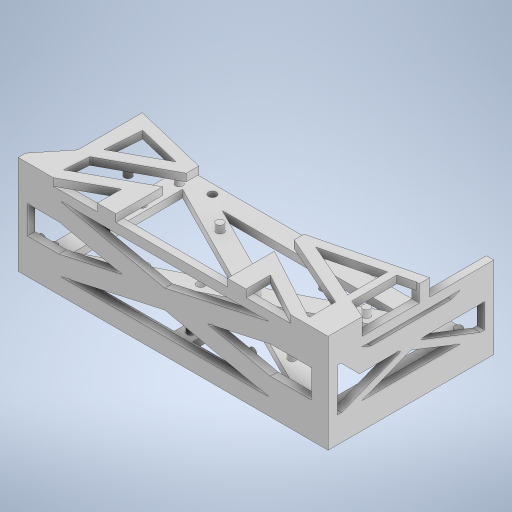
# Autodesk Inventor part: Power_Supply
Saved by Autodesk Inventor 2024 (Build 280153000, 153)
## iProperties
Created: 2024-11-22
Part Number: Power_Supply
Material: Generic
Document SubType Name: Modeling
Designer: Owner
Density: 1 g/cm^3
Appearance: Default
Author: Owner
Autodesk Inventor part; units mm, degrees
ref_plane "YZ Plane" through (0, 0, 0) normal (1, 0, 0) x (0, 1, 0)
ref_plane "XZ Plane" through (0, 0, 0) normal (0, 1, 0) x (-1, 0, 0)
ref_plane "XY Plane" through (0, 0, 0) normal (0, 0, 1) x (1, 0, 0)
sketch "Sketch1" plane through (0, 0, 0) normal (0, 1, 0) x (-1, 0, 0)
  line L0 (88.9, 50.8) -> (-88.9, 50.8)
  line L1 (-88.9, 50.8) -> (-88.9, -50.8)
  line L2 (-88.9, -50.8) -> (88.9, -50.8)
  line L3 (88.9, -50.8) -> (88.9, 50.8)
  line L4 (88.9, 50.8) -> (-88.9, -50.8) construction
  line L5 (-88.9, 50.8) -> (88.9, -50.8) construction
  point P0 (0, 0)
  dimension "d0" = 177.8
  dimension "d1" = 101.6
  constraints: 12 end point, 2 midpoint, 2 parallel, 1 horizontal, 1 perpendicular
  measures "d0" distance of L2.end L1.end
  measures "d1" distance of L1.end L0.end
extrude "Extrusion1" add sketch "Sketch1" along normal blind 44.45
sketch "Sketch2" plane through (-88.9, 0, 50.8) normal (0, 0, 1) x (1, 0, 0)
  line L0 (177.8, 0) -> (177.8, 44.45) projected
  line L1 (177.8, 44.45) -> (184.15, 44.45)
  line L2 (184.15, 44.45) -> (184.15, 0)
  line L3 (184.15, 0) -> (177.8, 0)
  line L4 (177.8, 0) -> (177.8, 44.45)
  line L5 (177.8, 44.45) -> (0, 44.45) projected
  line L6 (0, 44.45) -> (-15.875, 44.45)
  line L7 (-15.875, 44.45) -> (-15.875, 0)
  line L8 (-15.875, 0) -> (0, 0)
  line L9 (0, 0) -> (0, 44.45)
  point P0 (88.9, 0)
  dimension "d4" = 6.35
  dimension "d5" = 15.875
  constraints: 16 end point, 4 parallel, 2 horizontal, 2 perpendicular, 1 point on line
  measures "d4" distance of L2.end L3.end
  measures "d5" distance of L8.end L7.end
extrude "Extrusion2" add sketch "Sketch2" against normal blind 1.5875
sketch "Sketch3" plane through (0, 0, 0) normal (0, -1, 0) x (1, 0, 0)
  line L0 (-104.775, 49.2125) -> (-88.9, 49.2125) projected
  line L1 (-88.9, -50.8) -> (-88.9, 49.2125) projected
  line L2 (-104.775, 49.2125) -> (-88.9, 49.2125)
  line L3 (-88.9, 49.2125) -> (-88.9, -50.8)
  line L4 (-88.9, -50.8) -> (-104.775, -50.8)
  line L5 (-104.775, -50.8) -> (-104.775, 49.2125)
  line L6 (88.9, 49.2125) -> (95.25, 49.2125) projected
  line L7 (95.25, 49.2125) -> (88.9, 49.2125)
  line L8 (88.9, 49.2125) -> (88.9, -50.8)
  line L9 (88.9, -50.8) -> (95.25, -50.8)
  line L10 (95.25, -50.8) -> (95.25, 49.2125)
  point P0 (0, 0)
  constraints: 16 end point, 4 parallel, 2 horizontal, 2 perpendicular, 1 point on line
extrude "Extrusion3" add sketch "Sketch3" against normal blind 1.5875
sketch "Sketch4" plane through (0, 1.5875, 0) normal (0, 1, 0) x (1, 0, 0)
  line L0 (88.9, -49.2125) -> (95.25, -49.2125) projected
  line L1 (95.25, -50.8) -> (95.25, 50.8) projected
  line L2 (88.9, -49.2125) -> (95.25, -49.2125)
  line L3 (95.25, -49.2125) -> (95.25, 36.5125)
  line L4 (95.25, 36.5125) -> (88.9, 36.5125)
  line L5 (88.9, 36.5125) -> (88.9, -49.2125)
  point P0 (0, 0)
  dimension "d10" = 85.725
  constraints: 8 end point, 2 parallel, 1 horizontal, 1 perpendicular, 1 point on line
  measures "d10" distance of L3.end L2.end
extrude "Extrusion4" add sketch "Sketch4" along normal blind 12.7
sketch "Sketch5" plane through (-104.775, 0, 50.8) normal (0, 0, 1) x (1, 0, 0)
  line L0 (200.025, 44.45) -> (0, 44.45) projected
  line L1 (200.025, 0) -> (200.025, 44.45) projected
  line L2 (0, 44.45) -> (200.025, 0)
  line L3 (200.025, 0) -> (200.025, 44.45)
  line L4 (0, 0) -> (200.025, 0) projected
  line L5 (200.025, 44.45) -> (0, 0)
  line L6 (100.0125, 44.45) -> (100.0125, 0)
  line L7 (0, 44.45) -> (0, 0) projected
  line L8 (0, 22.225) -> (200.025, 22.225)
  line L9 (100.0125, 22.225) -> (0, 22.225)
  line L10 (100.0125, 22.225) -> (200.025, 22.225)
  line L11 (6.35, 6.35) -> (193.675, 6.35)
  line L12 (193.675, 6.35) -> (193.675, 38.1)
  line L13 (193.675, 38.1) -> (6.35, 38.1)
  line L14 (6.35, 38.1) -> (6.35, 6.35)
  line L15 (6.35, 6.35) -> (193.675, 38.1) construction
  line L16 (193.675, 6.35) -> (6.35, 38.1) construction
  circle A0 centre (6.35, 38.1) radius 2.54
  circle A1 centre (6.35, 6.35) radius 2.54
  circle A2 centre (100.0125, 22.225) radius 2.54
  circle A3 centre (193.675, 6.35) radius 2.54
  circle A4 centre (193.675, 38.1) radius 2.54
  line L17 (100.0125, 22.225) -> (0, 22.225)
  line L18 (50.0063, 22.225) -> (50.0063, 44.45)
  line L19 (50.0063, 22.225) -> (50.0063, 0)
  line L20 (100.0125, 22.225) -> (200.025, 22.225)
  line L21 (150.0188, 22.225) -> (150.0188, 44.45)
  line L22 (150.0188, 22.225) -> (150.0188, 0)
  circle A5 centre (50.0063, 33.3375) radius 2.54
  circle A6 centre (50.0063, 11.1125) radius 2.54
  circle A7 centre (150.0188, 11.1125) radius 2.54
  circle A8 centre (150.0188, 33.3375) radius 2.54
  point P0 (104.775, 0)
  dimension "d13" = 187.325
  dimension "d14" = 31.75
  dimension "d15" = 5.08
  dimension "d16" = 5.08
  dimension "d17" = 5.08
  dimension "d18" = 5.08
  dimension "d19" = 5.08
  dimension "d20" = 5.08
  dimension "d21" = 5.08
  dimension "d22" = 5.08
  dimension "d23" = 5.08
  constraints: 38 end point, 13 midpoint, 9 centre point, 6 point on line, 5 coincident, 4 collinear, 4 perpendicular, 2 parallel, 1 horizontal
  measures "d13" distance of L13.end L12.end
  measures "d14" distance of L12.end L11.end
  measures "d15" diameter of A0
  measures "d16" diameter of A1
  measures "d17" diameter of A2
  measures "d18" diameter of A3
  measures "d19" diameter of A4
  measures "d20" diameter of A5
  measures "d21" diameter of A6
  measures "d22" diameter of A7
  measures "d23" diameter of A8
extrude "Extrusion5" add sketch "Sketch5" along normal blind 6.35 contours A8 L21 L5 | L5 L21 A8 | A4 L12 L13 | L13 L12 A4 | L21 L5 A8 | A3 L11 L12 | L12 L11 A3 | L21 A8 L5 | A2 L5 L6 | L6 L2 A2 | A7 L22 L2 | L2 L22 A7 | A2 L2 L8 | L8 L5 A2 | L22 L2 A7 | A5 L2 L18 | L18 L2 A5 | L8 A2 L2 | L6 A2 L5 | L2 A2 L6 | L5 A2 L8 | L22 A7 L2 | L2 L18 A5 | A0 L14 L13 | L13 L14 A0 | L2 A5 L18 | A1 L11 L14 | L14 L11 A1 | A6 L19 L5 | L5 L19 A6 | A6 L5 L19 | A6 L19 L5
sketch "Sketch6" plane through (0, 44.45, 0) normal (0, 1, 0) x (1, 0, 0)
  line L0 (88.9, -49.2125) -> (88.9, 50.8) projected
  line L1 (88.9, 50.8) -> (-88.9, 50.8)
  line L2 (-88.9, 50.8) -> (-88.9, -50.8)
  line L3 (-88.9, -50.8) -> (88.9, -50.8)
  line L4 (88.9, -50.8) -> (88.9, 50.8)
  line L5 (-88.9, 0) -> (-88.9, -50.8)
  line L6 (-88.9, 0) -> (88.9, 0)
  line L7 (88.9, -50.8) -> (88.9, 0)
  line L8 (-88.9, 50.8) -> (-88.9, -49.2125) projected
  line L9 (-88.9, -25.4) -> (88.9, -25.4)
  line L10 (0, 0) -> (0, -50.8)
  line L11 (0, 0) -> (-88.9, 0)
  line L12 (0, 0) -> (88.9, 0)
  line L13 (-44.45, 0) -> (-44.45, -50.8)
  line L14 (44.45, 0) -> (44.45, -50.8)
  line L15 (-104.775, -50.8) -> (95.25, -50.8) projected
  line L16 (-88.9, 0) -> (88.9, -50.8)
  line L17 (-88.9, -50.8) -> (88.9, 0)
  circle A0 centre (-44.45, -12.7) radius 2.54
  circle A1 centre (44.45, -12.7) radius 2.54
  circle A2 centre (44.45, -38.1) radius 2.54
  circle A3 centre (-44.45, -38.1) radius 2.54
  line L18 (-88.9, -25.4) -> (-44.45, -25.4)
  circle A4 centre (-66.675, -25.4) radius 2.54
  line L19 (44.45, -25.4) -> (88.9, -25.4)
  circle A5 centre (66.675, -25.4) radius 2.54
  dimension "d26" = 5.08
  dimension "d27" = 5.08
  dimension "d28" = 5.08
  dimension "d29" = 5.08
  dimension "d30" = 5.08
  dimension "d31" = 5.08
  constraints: 34 end point, 11 point on line, 10 midpoint, 6 centre point, 3 collinear, 3 parallel, 3 perpendicular, 1 horizontal
  measures "d26" diameter of A0
  measures "d27" diameter of A1
  measures "d28" diameter of A2
  measures "d29" diameter of A3
  measures "d30" diameter of A4
  measures "d31" diameter of A5
extrude "Extrusion6" add sketch "Sketch6" along normal blind 6.35 contours A5 L9 | L9 A5 | A2 L14 L16 | L16 L14 A2 | A1 L14 L17 | L17 L14 A1 | A2 L16 L14 | L16 A2 L14 | L14 L17 A1 | L14 A1 L17 | A3 L17 L13 | L13 L17 A3 | A0 L13 L16 | L16 L13 A0 | L17 L13 A3 | A0 L13 L16 | L16 L13 A0 | A3 L13 L17 | A4 L9 | L9 A4
sketch "Sketch7" plane through (88.9, 44.45, 49.2125) normal (1, 0, 0) x (0, 0, -1)
  line L0 (0, -30.1625) -> (85.725, -30.1625) projected
  line L1 (85.725, -30.1625) -> (100.0125, -30.1625)
  line L2 (100.0125, -42.8625) -> (100.0125, 0) projected
  line L3 (0, 0) -> (100.0125, 0)
  line L4 (100.0125, 0) -> (100.0125, -30.1625)
  line L5 (100.0125, -30.1625) -> (0, -30.1625)
  line L6 (0, -30.1625) -> (0, 0)
  line L7 (0, -15.0813) -> (100.0125, -15.0813)
  line L8 (50.0062, 0) -> (50.0062, -30.1625)
  line L9 (50.0062, -15.0813) -> (0, -15.0813)
  line L10 (-1.5875, 0) -> (-1.5875, -44.45) projected
  line L11 (25.0031, -15.0813) -> (0, -15.0813)
  line L12 (12.5016, -15.0813) -> (12.5016, 0)
  line L13 (8.5725, 0) -> (13.6525, 0) projected
  line L14 (12.5016, -15.0813) -> (12.5016, -30.1625)
  line L15 (50.0062, -15.0813) -> (100.0125, -15.0813)
  line L16 (75.0094, -15.0813) -> (100.0125, -15.0813)
  line L17 (87.5109, -15.0813) -> (100.0125, -15.0813)
  line L18 (87.5109, -15.0813) -> (87.5109, 0)
  line L19 (87.5109, -15.0813) -> (87.5109, -30.1625)
  circle A0 centre (12.5016, -15.0813) radius 2.54
  circle A1 centre (50.0062, -15.0813) radius 2.54
  circle A2 centre (87.5109, -15.0813) radius 2.54
  point P0 (49.2125, -44.45)
  dimension "d34" = 5.08
  dimension "d35" = 5.08
  dimension "d36" = 5.08
  constraints: 32 end point, 9 midpoint, 7 point on line, 5 perpendicular, 3 centre point, 3 coincident, 3 collinear, 2 horizontal, 2 parallel
  measures "d34" diameter of A0
  measures "d35" diameter of A1
  measures "d36" diameter of A2
extrude "Extrusion7" add sketch "Sketch7" along normal blind 12.7 contours A0 L7 L14 | L14 L7 A0 | A0 L12 L7 | A1 L7 L8 | L8 L7 A1 | L12 A0 L7 | L8 A1 L7 | L7 A1 L8 | A2 L7 L19 | L19 L7 A2 | L18 A2 L7 | L7 A2 L18
sketch "Sketch8" plane through (-98.425, 6.35, 57.15) normal (0, 0, 1) x (1, 0, 0)
  line L0 (-6.35, 38.1) -> (9.525, 38.1) projected
  line L1 (-6.35, -6.35) -> (193.675, -6.35) projected
  line L2 (-6.35, 38.1) -> (193.675, 38.1)
  line L3 (193.675, 38.1) -> (193.675, -6.35)
  line L4 (193.675, -6.35) -> (-6.35, -6.35)
  line L5 (-6.35, -6.35) -> (-6.35, 38.1)
  line L6 (193.675, -6.35) -> (-6.35, 38.1)
  line L7 (193.675, 38.1) -> (-6.35, -6.35)
  line L8 (195.0525, 31.9012) -> (-4.9725, -12.5488)
  line L9 (192.2975, 44.2988) -> (-7.7275, -0.1512)
  line L10 (195.0525, -0.1512) -> (-4.9725, 44.2988)
  line L11 (192.2975, -12.5488) -> (-7.7275, 31.9012)
  point P0 (98.425, -6.35)
  point P1 (122.9346, 15.875)
  point P2 (193.675, 31.5951)
  point P3 (164.4029, 38.1)
  point P4 (93.6625, 22.3799)
  point P5 (22.9221, 38.1)
  point P6 (-6.35, 31.5951)
  point P7 (64.3904, 15.875)
  point P8 (-6.35, 0.1549)
  point P9 (22.9221, -6.35)
  point P10 (93.6625, 9.3701)
  point P11 (164.4029, -6.35)
  point P12 (193.675, 0.1549)
  dimension "d95" = 6.35
  dimension "d96" = 6.35
  dimension "d97" = 6.35
  dimension "d98" = 6.35
  constraints: 20 end point, 6 parallel, 1 horizontal, 1 perpendicular
  measures "d95" distance between parallel lines of L7 L8
  measures "d96" distance between parallel lines of L7 L9
  measures "d97" distance between parallel lines of L6 L10
  measures "d98" distance between parallel lines of L6 L11
extrude "Extrusion8" add sketch "Sketch8" along normal blind 5.08 contours L6 L9 L11 L5 | L0 L2 L10 L9 L6 | L9 L10 L7 L6 | L6 L7 L11 L9 | L9 L11 L7 L5 | L7 L10 L8 L6 | L6 L8 L11 L7 | L9 L2 L7 L10 | L7 L11 L8 L1 | L8 L10 L3 L6 | L6 L1 L11 L8 | L7 L3 L8 L10
sketch "Sketch9" plane through (101.6, 29.3688, -0.7937) normal (1, 0, 0) x (0, 0, -1)
  line L0 (-63.0237, 15.0813) -> (-63.0237, -29.3688) projected
  line L1 (-63.0237, 15.0813) -> (50.0063, 15.0813)
  line L2 (50.0063, 15.0813) -> (50.0063, -29.3688)
  line L3 (50.0063, -29.3688) -> (-63.0237, -29.3688)
  line L4 (-63.0237, -29.3688) -> (-63.0237, 15.0813)
  line L5 (50.0063, -29.3688) -> (-63.0237, 15.0813)
  line L6 (-63.0237, -29.3688) -> (-63.0237, 15.0813) projected
  line L7 (-63.0237, -29.3688) -> (50.0063, 15.0813)
  line L8 (-63.9533, -27.005) -> (49.0767, 17.445)
  line L9 (-62.0942, -31.7325) -> (50.9358, 12.7175)
  line L10 (49.0767, -31.7325) -> (-63.9533, 12.7175)
  line L11 (50.9358, -27.005) -> (-62.0942, 17.445)
  circle A0 centre (0, 0) radius 2.54 projected
  line L12 (0, 0) -> (50.0063, 0)
  line L13 (0, 0) -> (-63.0237, 0)
  line L14 (-63.0237, 6.35) -> (0, 6.35)
  line L15 (0, 6.35) -> (50.0063, 6.35)
  line L16 (-63.0237, -6.35) -> (0, -6.35)
  line L17 (0, -6.35) -> (50.0063, -6.35)
  line L18 (43.6563, 8.7312) -> (-56.6737, 8.7312)
  line L19 (-56.6737, 8.7312) -> (-56.6737, -23.0187)
  line L20 (-56.6737, -23.0187) -> (43.6563, -23.0187)
  line L21 (43.6563, -23.0187) -> (43.6563, 8.7312)
  line L22 (43.6563, 8.7312) -> (-56.6737, -23.0187) construction
  line L23 (-56.6737, 8.7312) -> (43.6563, -23.0187) construction
  line L24 (-56.6737, 8.7312) -> (-41.5925, -6.35)
  line L25 (-56.6737, 8.7312) -> (-35.3456, 8.7312) construction
  point P0 (-0.7937, -29.3688)
  point P1 (-6.5087, -7.1437)
  point P2 (-39.9363, -23.0187)
  point P3 (-6.5087, -9.8731)
  point P4 (26.9188, -23.0187)
  point P5 (-15.4675, -6.35)
  point P6 (-13.4491, -7.1437)
  point P7 (-53.817, -23.0187)
  point P8 (-56.6737, 6.35)
  point P9 (-54.2925, 6.35)
  point P10 (0.4316, -7.1437)
  point P11 (2.45, -6.35)
  point P12 (43.6563, -6.35)
  point P13 (40.7995, -23.0187)
  point P14 (-33.8811, 6.35)
  point P15 (-39.9363, 8.7312)
  point P16 (26.9188, 8.7312)
  point P17 (20.8636, 6.35)
  dimension "d86" = 2.54
  dimension "d87" = 2.54
  dimension "d88" = 2.54
  dimension "d89" = 2.54
  dimension "d90" = 6.35
  dimension "d91" = 6.35
  dimension "d92" = 100.33
  dimension "d93" = 31.75
  dimension "d94" = 45
  constraints: 48 end point, 8 parallel, 4 point on line, 3 horizontal, 3 midpoint, 3 perpendicular, 1 equal length, 2 other
  measures "d86" distance between parallel lines of L7 L8
  measures "d87" distance between parallel lines of L7 L9
  measures "d88" distance between parallel lines of L5 L10
  measures "d89" distance between parallel lines of L5 L11
  measures "d90" distance between parallel lines of L13 L14
  measures "d91" distance between parallel lines of L13 L16
  measures "d92" distance of L20.end L19.end
  measures "d93" distance of L19.end L18.end
  measures "d94" angle of L24 L25
extrude "Extrusion9" add sketch "Sketch9" along normal blind 5.08 contours L14 L19 L13 L0 | L0 L10 L18 L19 L14 | L13 L19 L16 L0 | L0 L5 L18 L10 | L19 L24 L14 | L16 L19 L20 L8 L0 | L1 L11 L18 L5 | L18 L5 L14 L10 | L10 L14 L24 L18 | L14 L10 L13 L24 | L8 L20 L7 L0 | L13 L10 L16 L24 | L1 L8 L18 L11 | L18 L11 L14 L5 | L14 L5 L13 L10 | L7 L20 L9 L3 | L8 L10 L7 L20 | L13 L5 L8 L16 L10 | L1 L7 L18 L8 | L14 L11 L13 L5 | L9 L20 L10 L3 | L7 L10 L9 L20 | L10 L16 L8 | L8 L16 L5 L7 L10 | L13 L11 L8 L5 | L2 L9 L18 L7 | L18 L7 L15 L8 | L14 L15 L8 L12 A0 L13 L11 | L10 L20 L5 L3 | L7 L5 L9 L10 | L8 L5 L16 | L8 L11 L7 L16 L5 | L13 A0 L8 L11 | L2 L15 L21 L18 L9 | L18 L9 L15 L7 | L15 L7 L12 L8 | L5 L20 L11 L2 | L10 L9 L5 L20 | L7 L16 L11 L9 L5 | L5 L16 L7 | L8 A0 L12 L7 L11 | L13 L12 A0 L8 | A0 L12 L13 | L2 L12 L21 L15 | L18 L21 L15 L9 | L15 L9 L12 L7 | L8 A0 L12 | L11 L20 L21 L17 L2 | L5 L9 L11 L20 | L7 L11 L16 | L8 A0 | L7 L12 L9 L17 L16 L11 | L2 L17 L21 L12 | L21 L12 L9 L15 | L11 L16 L17 L9 | L21 L17 L9 L12
sketch "Sketch10" plane through (-44.45, 50.8, 12.7) normal (0, 1, 0) x (1, 0, 0)
  line L0 (151.13, 63.5) -> (151.13, -49.53) projected
  line L1 (-60.325, -44.45) -> (-60.325, -49.53) projected
  line L2 (151.13, 63.5) -> (-60.325, 63.5)
  line L3 (-60.325, 63.5) -> (-60.325, -49.53)
  line L4 (-60.325, -49.53) -> (151.13, -49.53)
  line L5 (151.13, -49.53) -> (151.13, 63.5)
  line L6 (-60.325, -38.1) -> (-60.325, 63.5) projected
  line L7 (-60.325, 12.7) -> (151.13, 12.7)
  line L8 (151.13, 12.7) -> (151.13, -49.53)
  line L9 (151.13, -49.53) -> (-60.325, -49.53)
  line L10 (-60.325, -49.53) -> (-60.325, 12.7)
  line L11 (-44.45, 63.5) -> (-44.45, -36.5125) projected
  circle A0 centre (0, 0) radius 2.54 projected
  line L12 (0, 0) -> (6.333, 0.4643)
  line L13 (6.333, 0.4643) -> (6.333, 12.7)
  line L14 (6.333, 0.4643) -> (6.333, -49.53)
  line L15 (-44.45, 12.7) -> (6.333, 0.4643)
  line L16 (133.35, -36.5125) -> (133.35, 49.2125) projected
  circle A1 centre (88.9, 0) radius 2.54 projected
  line L17 (88.9, 0) -> (82.55, 0)
  line L18 (82.55, 0) -> (82.55, 12.7)
  line L19 (82.55, 0) -> (82.55, -38.1)
  line L20 (82.55, -38.1) -> (133.35, -38.1)
  line L21 (82.55, -38.1) -> (133.35, -38.1)
  line L22 (151.13, 17.145) -> (82.55, 0)
  line L23 (-44.224, 15.2582) -> (6.6826, 2.9927)
  line L24 (151.13, 19.7632) -> (81.934, 2.4642)
  line L25 (-44.45, 12.7) -> (-44.45, -49.53)
  line L26 (-44.45, -49.53) -> (6.333, -49.53)
  line L27 (82.55, -38.1) -> (82.55, -49.53)
  line L28 (82.55, -49.53) -> (151.13, -49.53)
  line L29 (6.6826, 2.9927) -> (-44.45, -24.765)
  circle A2 centre (0, -25.4) radius 2.54 projected
  line L30 (-44.45, -49.53) -> (0, -25.4)
  line L31 (0, -25.4) -> (6.333, -21.9621)
  line L32 (-46.2677, -21.4166) -> (-3.8484, 1.6111)
  line L33 (-3.8484, 1.6111) -> (-45.1165, 11.5542)
  line L34 (-44.45, -29.1002) -> (17.2137, 4.3744)
  line L35 (17.2137, 4.3744) -> (-44.45, 19.2317)
  line L36 (-46.2677, -46.1816) -> (6.333, -17.6269)
  line L37 (-1.8177, -22.0516) -> (4.5153, -18.6137)
  line L38 (-42.6323, -52.8784) -> (1.8177, -28.7484)
  line L39 (1.8177, -28.7484) -> (8.1507, -25.3105)
  line L40 (0, -25.4) -> (-6.35, -25.4)
  line L41 (-6.35, -25.4) -> (-6.35, -49.53)
  circle A3 centre (111.125, -12.7) radius 2.54 projected
  line L42 (82.55, 0) -> (111.125, -12.7)
  line L43 (111.125, -12.7) -> (151.13, -30.48)
  line L44 (84.0974, 3.4816) -> (112.6724, -9.2184)
  line L45 (112.6724, -9.2184) -> (152.6774, -26.9984)
  line L46 (151.13, -34.6493) -> (109.5776, -16.1816)
  line L47 (109.5776, -16.1816) -> (81.0026, -3.4816)
  line L48 (-60.325, -49.53) -> (-44.45, -24.765)
  line L49 (-44.45, -49.53) -> (-38.1, -49.53)
  line L50 (-38.1, -49.53) -> (-33.6063, 12.7)
  circle A4 centre (88.9, -25.4) radius 2.54 projected
  line L51 (82.55, -21.9621) -> (88.9, -25.4)
  line L52 (88.9, -25.4) -> (133.4693, -49.53)
  line L53 (141.4717, -49.53) -> (90.714, -22.0495)
  line L54 (90.714, -22.0495) -> (82.55, -17.6295)
  line L55 (131.6553, -52.8805) -> (87.086, -28.7505)
  line L56 (87.086, -28.7505) -> (80.736, -25.3126)
  line L57 (152.0541, 13.4488) -> (83.4741, -3.6962)
  line L58 (146.05, -49.53) -> (151.13, -49.53) projected
  line L59 (151.13, -49.53) -> (138.43, -49.53)
  line L60 (138.43, -49.53) -> (138.43, 12.7)
  line L61 (133.4693, -49.53) -> (133.35, 12.7)
  line L62 (88.9, -25.4) -> (95.25, -25.4)
  line L63 (68.9596, -44.45) -> (131.7015, -44.45) projected
  line L64 (95.25, -25.4) -> (95.25, -49.53)
  line L65 (-44.45, 19.2317) -> (-44.45, 12.7)
  point P0 (44.45, 12.7)
  point P1 (6.333, 2.8029)
  point P2 (6.333, 3.077)
  point P3 (6.333, 6.996)
  point P4 (-17.3409, 12.7)
  point P5 (-36.4641, -49.53)
  point P6 (-6.35, -33.1823)
  point P7 (-6.35, -49.53)
  point P8 (-44.45, -45.1948)
  point P9 (-44.45, -36.5125)
  point P10 (6.333, -1.5323)
  point P11 (-44.45, -20.4298)
  point P12 (-44.45, 11.3937)
  point P13 (133.35, -18.4084)
  point P14 (94.2091, -1.0125)
  point P15 (133.35, 8.7727)
  point P16 (82.55, -4.1693)
  point P17 (138.43, -29.0049)
  point P18 (138.43, -47.8832)
  point P19 (82.55, -49.53)
  point P20 (82.55, 2.6182)
  point P21 (133.4257, -26.7808)
  point P22 (133.461, -45.1929)
  point P23 (95.25, -49.53)
  point P24 (95.25, -33.1705)
  point P25 (125.4668, -49.53)
  point P26 (151.13, -26.3107)
  point P27 (138.43, -20.6662)
  point P28 (138.43, 10.0427)
  point P29 (149.059, 12.7)
  point P30 (-37.5151, -41.4301)
  point P31 (-36.3055, -24.6789)
  point P32 (-35.6539, -15.6548)
  point P33 (-33.8845, 8.848)
  dimension "d106" = 6.35
  dimension "d107" = 6.35
  dimension "d108" = 2.54
  dimension "d109" = 2.54
  dimension "d110" = 3.81
  dimension "d111" = 3.81
  dimension "d112" = 3.81
  dimension "d113" = 3.81
  dimension "d114" = 6.35
  dimension "d115" = 3.81
  dimension "d116" = 3.81
  dimension "d117" = 6.35
  dimension "d118" = 3.81
  dimension "d119" = 3.81
  dimension "d120" = 3.81
  dimension "d121" = 12.7
  dimension "d122" = 6.35
  constraints: 118 end point, 33 point on line, 10 perpendicular, 9 parallel, 4 collinear, 4 horizontal, 1 midpoint, 4 other
  measures "d106" distance of L12.start L12.end
  measures "d107" distance of L17.start L17.end
  measures "d108" distance between parallel lines of L15 L23
  measures "d109" distance between parallel lines of L22 L24
  measures "d110" distance between parallel lines of L29 L32
  measures "d111" distance between parallel lines of L29 L34
  measures "d112" distance between parallel lines of L30 L36
  measures "d113" distance between parallel lines of L30 L38
  measures "d114" distance of L30.end L40.end
  measures "d115" distance between parallel lines of L42 L44
  measures "d116" distance between parallel lines of L43 L46
  measures "d117" distance of L25.end L49.end
  measures "d118" distance between parallel lines of L52 L53
  measures "d119" distance between parallel lines of L52 L55
  measures "d120" distance between parallel lines of L22 L57
  measures "d121" distance of L0.end L59.end
  measures "d122" distance of L51.end L62.end
extrude "Extrusion10" add sketch "Sketch10" along normal blind 5.08 contours L0 L22 L16 L24 | L0 L57 L7 L22 | L16 L7 L24 | L35 L7 L11 | L0 L7 L57 | L22 A1 L44 L24 L7 | L61 L57 L16 | L16 L57 L44 A1 L22 | L7 L60 L57 L61 | L15 L50 L33 L11 | L7 L50 L15 | L35 L13 L23 L7 | L57 L60 L7 | L57 L61 L45 L16 | L22 L44 A1 | A1 L44 L22 | L57 L60 L45 L61 | L44 A1 L22 L18 L24 | L23 L13 L29 L15 A0 L50 | L33 L50 L32 L11 | L15 A0 L29 L50 L32 L33 | L0 L43 L60 L45 | L45 L61 L43 L16 | L16 L43 A3 L42 L57 A1 L44 L45 | L57 A1 L44 | A1 L57 L22 L44 | L44 L22 A1 | L45 L60 L43 L61 | L32 L50 L29 L11 | L15 A0 L29 | A0 L15 | L0 L46 L60 L43 | L43 L61 L46 L16 | L16 L46 L47 L19 L42 A3 L43 | A1 L57 | A1 L17 L22 | L43 L60 L46 L61 | L17 A1 L57 L42 | L48 L11 L25 L4 | L13 L15 L29 | L29 L50 L34 L11 | L15 L29 A0 | L29 L12 A0 | A0 L12 L14 L34 L50 L29 | L0 L4 L53 L60 L46 | L43 L42 A3 | A3 L42 L43 | L46 L60 L53 L61 | L30 L50 L4 | L25 L36 L50 L30 | L12 A0 L29 L15 | L34 L50 L36 L25 L11 | A0 L12 L29 | L14 L31 A2 L40 L41 L30 L50 L36 | L61 L52 L20 L53 | L53 L60 L4 L61 | L54 L53 L20 L52 L64 L62 A4 L51 L19 | L50 L30 L41 L38 L4 | L14 L39 L38 L41 L30 A2 L31 | L53 L4 L60 | L4 L55 L63 L52 | L51 A4 L52 L64 L55 L56 L19 | L41 L40 A2 L30 | L14 L4 L41 L38 L39 | L31 L40 A2 | A2 L30 L31 | L52 L63 L55 L20 | L20 L55 L64 L52 | L56 L55 L64 L20 L19 | L51 L52 A4 | A4 L62 L51 | A2 L40 L30 | L52 A4 L62 L64 | L4 L27 L63 L64 | L20 L64 L63 L27 | A4 L52 L62
sketch "Sketch11" plane through (-104.775, 0, 57.15) normal (-1, 0, 0) x (0, 0, 1)
  line L0 (0, 0) -> (0, 44.45) projected
  line L1 (0, 44.45) -> (0, 50.8)
  line L2 (5.08, 50.8) -> (-64.2132, 50.8) projected
  line L3 (-107.95, 44.45) -> (5.08, 44.45) projected
  line L4 (0, 50.8) -> (5.08, 50.8)
  line L5 (5.08, 50.8) -> (5.08, 44.45)
  line L6 (5.08, 44.45) -> (0, 44.45)
  line L7 (0, 44.45) -> (0, 50.8)
  point P0 (-57.15, 0)
  point P1 (-57.15, 50.8)
  constraints: 10 end point, 2 parallel, 1 horizontal, 1 perpendicular, 1 point on line, 1 vertical
extrude "Extrusion11" add sketch "Sketch11" against normal up to surface (211.455 mm away)
sketch "Sketch12" plane through (101.6, 44.45, 57.15) normal (0, -1, 0) x (1, 0, 0)
  line L0 (-6.35, 0) -> (-6.35, 5.08) projected
  line L1 (-6.35, 5.08) -> (0, 5.08) projected
  line L2 (-6.35, 0) -> (0, 0)
  line L3 (0, 0) -> (0, 5.08)
  line L4 (0, 5.08) -> (-6.35, 5.08)
  line L5 (-6.35, 5.08) -> (-6.35, 0)
  point P0 (-101.6, -57.15)
  constraints: 8 end point, 2 parallel, 1 horizontal, 1 perpendicular
extrude "Extrusion12" add sketch "Sketch12" along normal up to surface (44.45 mm away)
sketch "Sketch13" plane through (-98.425, 6.35, 57.15) normal (0, 0, -1) x (-1, 0, 0)
  line L0 (-200.025, 38.1) -> (-205.105, 38.1) projected
  line L1 (-200.025, 38.1) -> (-200.025, 44.45)
  line L2 (-205.105, 44.45) -> (3.0936, 44.45) projected
  line L3 (-205.105, 44.45) -> (-205.105, 38.1) projected
  line L4 (-200.025, 44.45) -> (-205.105, 44.45)
  line L5 (-205.105, 44.45) -> (-205.105, 38.1)
  line L6 (-205.105, 38.1) -> (-200.025, 38.1)
  line L7 (-200.025, 38.1) -> (-200.025, 44.45)
  point P0 (-98.425, -6.35)
  point P1 (6.35, 44.45)
  constraints: 10 end point, 2 parallel, 1 horizontal, 1 perpendicular, 1 point on line, 1 vertical
extrude "Extrusion13" add sketch "Sketch13" along normal up to surface (57.15 mm away)
sketch "Sketch14" plane through (0, 0, 0) normal (0, -1, 0) x (1, 0, 0)
  line L0 (95.25, 50.8) -> (95.25, -50.8) projected
  line L1 (95.25, 50.8) -> (-104.775, 50.8) projected
  line L2 (95.25, -50.8) -> (-104.775, -50.8)
  line L3 (-104.775, -50.8) -> (-104.775, 50.8)
  line L4 (-104.775, 50.8) -> (95.25, 50.8)
  line L5 (95.25, 50.8) -> (95.25, -50.8)
  line L6 (-104.775, -50.8) -> (95.25, -50.8) projected
  line L7 (-4.7625, -50.8) -> (-4.7625, 50.8)
  line L8 (104.609, 0) -> (106.68, 0) projected
  line L9 (95.25, 0) -> (-104.775, 0)
  line L10 (88.9, 44.45) -> (-98.425, 44.45)
  line L11 (-98.425, 44.45) -> (-98.425, -44.45)
  line L12 (-98.425, -44.45) -> (88.9, -44.45)
  line L13 (88.9, -44.45) -> (88.9, 44.45)
  line L14 (88.9, 44.45) -> (-98.425, -44.45) construction
  line L15 (-98.425, 44.45) -> (88.9, -44.45) construction
  line L16 (95.25, -50.8) -> (-104.775, 50.8)
  line L17 (95.25, 50.8) -> (-104.775, -50.8)
  line L18 (95.25, 0) -> (-4.7625, 0)
  line L19 (45.2438, 0) -> (45.2438, -50.8)
  line L20 (45.2438, 0) -> (45.2438, 44.45)
  line L21 (-4.7625, 0) -> (-104.775, 0)
  line L22 (-54.7688, 0) -> (-54.7688, -44.45)
  line L23 (-54.7688, 0) -> (-54.7688, 50.8)
  circle A0 centre (-4.7625, 0) radius 2.54
  circle A1 centre (-54.7688, -25.4) radius 2.54
  circle A2 centre (-54.7688, 25.4) radius 2.54
  circle A3 centre (45.2438, 25.4) radius 2.54
  circle A4 centre (45.2438, -25.4) radius 2.54
  circle A5 centre (88.9, -44.45) radius 2.54
  circle A6 centre (88.9, 44.45) radius 2.54
  circle A7 centre (-98.425, 44.45) radius 2.54
  circle A8 centre (-98.425, -44.45) radius 2.54
  circle A9 centre (-4.7625, 44.45) radius 2.54
  circle A10 centre (-4.7625, -44.45) radius 2.54
  point P0 (0, 0)
  point P1 (101.6, 0)
  point P2 (-4.7625, 46.99)
  point P3 (-4.7625, 44.45)
  point P4 (-7.3025, 44.45)
  point P5 (-61.7909, 0)
  dimension "d51" = 187.325
  dimension "d52" = 88.9
  dimension "d53" = 5.08
  dimension "d54" = 5.08
  dimension "d55" = 5.08
  dimension "d56" = 5.08
  dimension "d57" = 5.08
  dimension "d58" = 5.08
  dimension "d59" = 5.08
  dimension "d60" = 5.08
  dimension "d61" = 5.08
  dimension "d62" = 5.08
  dimension "d63" = 5.08
  constraints: 40 end point, 12 midpoint, 11 centre point, 10 point on line, 5 coincident, 4 parallel, 4 perpendicular, 3 collinear, 2 horizontal
  measures "d51" distance of L12.end L11.end
  measures "d52" distance of L11.end L10.end
  measures "d53" diameter of A0
  measures "d54" diameter of A1
  measures "d55" diameter of A2
  measures "d56" diameter of A3
  measures "d57" diameter of A4
  measures "d58" diameter of A5
  measures "d59" diameter of A6
  measures "d60" diameter of A7
  measures "d61" diameter of A8
  measures "d62" diameter of A9
  measures "d63" diameter of A10
extrude "Extrusion14" add sketch "Sketch14" along normal blind 6.35 contours A9 L10 L7 | L7 L10 A9 | A6 L13 L10 | L10 L13 A6 | A3 L20 L17 | L17 L20 A3 | A5 L12 L13 | L13 L12 A5 | L10 A9 L7 | L7 A9 L10 | L20 L17 A3 | L20 A3 L17 | A4 L19 L16 | L16 L19 A4 | A0 L16 L9 | L9 L17 A0 | L19 L16 A4 | A2 L16 L23 | L23 L16 A2 | A10 L12 L7 | L7 L12 A10 | L12 L7 A10 | A4 L16 L19 | L16 A0 L7 | L16 A0 L7 | L17 A0 L9 | L9 A0 L16 | L7 A0 L17 | L7 A0 L17 | A7 L11 L10 | L10 L11 A7 | L16 L23 A2 | L16 A2 L23 | L12 A10 L7 | A8 L12 L11 | L11 L12 A8 | A1 L22 L17 | L17 L22 A1 | A1 L22 L17 | L17 L22 A1
sketch "Sketch15" plane through (88.9, -6.35, -44.45) normal (0, -1, 0) x (1, 0, 0)
  line L0 (-193.675, 106.68) -> (17.78, 106.68) projected
  line L1 (-193.675, 106.68) -> (17.78, 106.68)
  line L2 (17.78, 106.68) -> (17.78, -6.35)
  line L3 (17.78, -6.35) -> (-193.675, -6.35)
  line L4 (-193.675, -6.35) -> (-193.675, 106.68)
  line L5 (0, -6.35) -> (-6.35, -6.35)
  line L6 (0, -6.35) -> (-177.8, -6.35) projected
  line L7 (-6.35, -6.35) -> (17.78, -6.35)
  line L8 (17.78, -6.35) -> (17.78, 106.68)
  line L9 (17.78, 106.68) -> (-6.35, 106.68)
  line L10 (-6.35, 106.68) -> (-6.35, -6.35)
  line L11 (-193.675, -6.35) -> (6.35, -6.35) projected
  line L12 (-193.675, -6.35) -> (-180.975, -6.35)
  line L13 (-180.975, -6.35) -> (-180.975, 106.68)
  line L14 (-180.975, 106.68) -> (-193.675, 106.68)
  line L15 (-193.675, 106.68) -> (-193.675, -6.35)
  line L16 (6.35, -6.35) -> (-193.675, 95.25)
  line L17 (6.35, 95.25) -> (-193.675, -6.35)
  line L18 (3.4743, -12.0115) -> (-196.5507, 89.5885)
  line L19 (9.2257, -0.6885) -> (-190.7993, 100.9115)
  line L20 (9.2257, 89.5885) -> (-190.7993, -12.0115)
  line L21 (3.4743, 100.9115) -> (-196.5507, -0.6885)
  line L22 (17.78, 106.68) -> (-193.675, 106.68)
  line L23 (-193.675, 106.68) -> (-193.675, 93.98)
  line L24 (-193.675, 93.98) -> (17.78, 93.98)
  line L25 (17.78, 93.98) -> (17.78, 106.68)
  line L26 (17.78, -6.35) -> (-193.675, -6.35)
  line L27 (-193.675, -6.35) -> (-193.675, 6.35)
  line L28 (-193.675, 6.35) -> (17.78, 6.35)
  line L29 (17.78, 6.35) -> (17.78, -6.35)
  point P0 (-88.9, 44.45)
  point P1 (-79.6407, 44.45)
  point P2 (-6.35, 81.677)
  point P3 (-6.35, 7.223)
  point P4 (-93.6625, 37.3278)
  point P5 (-32.6749, 6.35)
  point P6 (-154.6501, 6.35)
  point P7 (-107.6843, 44.45)
  point P8 (-180.975, 7.223)
  point P9 (-180.975, 81.677)
  point P10 (-10.1721, 93.98)
  point P11 (-93.6625, 51.5722)
  point P12 (-177.1529, 93.98)
  dimension "d72" = 6.35
  dimension "d73" = 12.7
  dimension "d74" = 6.35
  dimension "d75" = 6.35
  dimension "d76" = 6.35
  dimension "d77" = 6.35
  dimension "d78" = 12.7
  dimension "d79" = 12.7
  constraints: 54 end point, 14 parallel, 5 horizontal, 5 perpendicular, 5 point on line
  measures "d72" distance of L5.start L5.end
  measures "d73" distance of L14.end L13.end
  measures "d74" distance between parallel lines of L16 L18
  measures "d75" distance between parallel lines of L16 L19
  measures "d76" distance between parallel lines of L17 L20
  measures "d77" distance between parallel lines of L17 L21
  measures "d78" distance of L23.end L22.end
  measures "d79" distance of L26.end L27.end
extrude "Extrusion15" add sketch "Sketch15" along normal blind 5.08 contours L0 L13 L24 L16 L4 | L0 L10 L21 L24 L19 L13 | L16 L24 L4 | L0 L2 L24 L10 | L19 L24 L13 | L24 L16 L13 L18 L4 | L24 L13 L16 | L10 L24 L21 | L24 L19 L21 L16 L13 | L18 L13 L21 L28 L4 | L16 L21 L18 L13 | L2 L28 L19 L10 L17 L24 | L24 L17 L10 | L10 L17 L19 L21 L24 | L19 L17 L16 L21 | L28 L21 L4 | L16 L17 L18 L21 | L2 L3 L16 L10 L28 | L10 L20 L19 L17 | L19 L20 L16 L17 | L21 L28 L13 L17 L4 | L21 L13 L28 | L21 L18 L17 L28 L13 | L16 L20 L18 L17 | L28 L10 L19 | L19 L10 L28 L16 L20 | L17 L13 L3 | L28 L17 L13 | L18 L20 L28 L17 | L16 L28 L18 L20 | L3 L10 L16 | L10 L16 L28 | L13 L17 L28 L20 L3 | L16 L10 L3 L18 L28 | L20 L28 L18 L3
sketch "Sketch16" plane through (106.68, -6.35, 62.23) normal (1, 0, 0) x (0, 0, -1)
  line L0 (0, 6.35) -> (0, 62.23) projected
  line L1 (113.03, 0) -> (0, 0) projected
  line L2 (0, 6.35) -> (113.03, 6.35)
  line L3 (113.03, 6.35) -> (113.03, 0)
  line L4 (113.03, 0) -> (0, 0)
  line L5 (0, 0) -> (0, 6.35)
  point P0 (62.23, 6.35)
  constraints: 8 end point, 2 parallel, 1 horizontal, 1 perpendicular
extrude "Extrusion16" add sketch "Sketch16" against normal up to surface (5.08 mm away)
sketch "Sketch17" plane through (101.6, 29.3688, -0.7937) normal (-1, 0, 0) x (0, 0, 1)
  line L0 (57.9437, -29.3688) -> (63.0237, -29.3688) projected
  line L1 (57.9437, -29.3688) -> (57.9437, -35.7188)
  line L2 (63.0238, -35.7188) -> (-50.0063, -35.7188) projected
  line L3 (63.0238, -35.7188) -> (63.0237, -29.3688) projected
  line L4 (57.9437, -29.3688) -> (63.0238, -29.3688)
  line L5 (63.0238, -29.3688) -> (63.0238, -35.7188)
  line L6 (63.0238, -35.7188) -> (57.9437, -35.7188)
  line L7 (57.9437, -35.7188) -> (57.9437, -29.3688)
  point P0 (0.7937, -29.3688)
  constraints: 10 end point, 2 parallel, 1 horizontal, 1 perpendicular, 1 point on line, 1 vertical
extrude "Extrusion17" add sketch "Sketch17" along normal up to surface (206.375 mm away)
sketch "Sketch18" plane through (88.9, -11.43, -44.45) normal (0, -1, 0) x (1, 0, 0)
  circle A0 centre (-93.6625, 88.9) radius 2.54 projected
  line L0 (-93.6625, 88.9) -> (-93.6625, 93.98)
  line L1 (-177.1529, 93.98) -> (-10.1721, 93.98) projected
  line L2 (-93.6625, 93.98) -> (-87.3125, 93.98)
  line L3 (-93.6625, 88.9) -> (-93.6625, 82.55)
  line L4 (-93.6625, 82.55) -> (-100.0125, 82.55)
  line L5 (-87.3125, 93.98) -> (-100.0125, 93.98)
  line L6 (-100.0125, 93.98) -> (-100.0125, 82.55)
  line L7 (-100.0125, 82.55) -> (-87.3125, 82.55)
  line L8 (-87.3125, 82.55) -> (-87.3125, 93.98)
  point P0 (-88.9, 44.45)
  dimension "d80" = 6.35
  dimension "d81" = 6.35
  dimension "d82" = 6.35
  constraints: 16 end point, 2 parallel, 2 perpendicular, 1 horizontal, 1 midpoint, 1 point on line, 1 vertical
  measures "d80" distance of L0.end L2.end
  measures "d81" distance of L0.start L3.end
  measures "d82" distance of L3.end L4.end
extrude "Extrusion18" add sketch "Sketch18" against normal up to surface (5.08 mm away)
fillet "Fillet1" radius 3.175 2 edges at (-11.1125, -8.89, 38.1) (1.5875, -8.89, 38.1)
sketch "Sketch19" plane through (-104.775, 0, 57.15) normal (0, 0, 1) x (1, 0, 0)
  circle A0 centre (193.675, 38.1) radius 2.54 projected
  line L0 (193.675, 38.1) -> (193.675, 31.75)
  line L1 (193.675, 44.45) -> (193.675, 14.2875) projected
  circle A1 centre (193.675, 6.35) radius 2.54 projected
  line L2 (193.675, 6.35) -> (193.675, 12.7)
  line L3 (193.675, 1.5875) -> (193.675, 44.45) projected
  line L4 (193.675, 12.7) -> (200.025, 12.7)
  line L5 (200.025, 1.5875) -> (200.025, 14.2875) projected
  line L6 (193.675, 12.7) -> (172.1471, 12.7)
  line L7 (192.0265, 8.2824) -> (129.2846, 22.225) projected
  line L8 (193.675, 31.75) -> (200.025, 31.75)
  line L9 (200.025, 31.75) -> (172.1471, 31.75)
  line L10 (129.2846, 22.225) -> (200.025, 37.9451) projected
  line L11 (172.1471, 31.75) -> (200.025, 37.9451)
  line L12 (200.025, 37.9451) -> (200.025, 31.75)
  line L13 (200.025, 6.5049) -> (129.2846, 22.225) projected
  line L14 (172.1471, 12.7) -> (200.025, 6.5049)
  line L15 (200.025, 6.5049) -> (200.025, 12.7)
  circle A2 centre (6.35, 38.1) radius 2.54 projected
  line L16 (6.35, 38.1) -> (6.35, 31.75)
  line L17 (6.35, 31.75) -> (0, 31.75)
  line L18 (0, 44.45) -> (0, 0) projected
  line L19 (0, 38.1) -> (0, 31.75)
  line L20 (6.35, 31.75) -> (27.8779, 31.75)
  line L21 (7.9985, 36.1676) -> (70.7404, 22.225) projected
  line L22 (0, 37.9451) -> (4.0382, 37.0477) projected
  line L23 (0, 37.9451) -> (27.8779, 31.75)
  circle A3 centre (6.35, 6.35) radius 2.54 projected
  line L24 (6.35, 6.35) -> (6.35, 12.7)
  line L25 (6.35, 12.7) -> (0, 12.7)
  line L26 (0, 12.7) -> (27.8779, 12.7)
  line L27 (27.8779, 12.7) -> (0, 6.5049)
  line L28 (0, 6.5049) -> (0, 12.7)
  point P0 (104.775, 0)
  dimension "d99" = 6.35
  dimension "d100" = 6.35
  dimension "d101" = 6.35
  dimension "d102" = 6.35
  constraints: 40 end point, 17 point on line, 4 collinear, 3 perpendicular, 1 horizontal, 1 parallel, 1 other
  measures "d99" distance of L0.start L0.end
  measures "d100" distance of L2.start L2.end
  measures "d101" distance of L16.start L16.end
  measures "d102" distance of L24.start L24.end
extrude "Extrusion19" add sketch "Sketch19" along normal blind 5.08 contours L10 L12 L8 L0 A0 | A0 L0 L10 | L10 L0 A0 | A0 L0 L9 L10 | L6 L2 A1 L7 | L4 L5 L13 A1 L2 | A1 L2 L13 | A1 L13 L2 | L23 L16 A2 | A2 L16 L17 L18 L22 | L21 L20 L16 A2 | A2 L16 L23 | L25 L24 A3 L27 L18 | L26 L27 A3 L24 | A3 L24 L27 | A3 L27 L24
sketch "Sketch20" plane through (106.68, 50.8, -7.0632) normal (1, 0, 0) x (0, 0, -1)
  line L0 (0, 0) -> (-17.145, 0) projected
  line L1 (43.7368, -6.35) -> (-56.2757, -6.35) projected
  line L2 (0, 0) -> (-7.0632, 0)
  line L3 (-7.0632, 0) -> (-7.0632, -6.35)
  line L4 (-7.0632, -6.35) -> (0, -6.35)
  line L5 (0, -6.35) -> (0, 0)
  point P0 (-7.0632, -50.8)
  point P1 (0, -6.35)
  constraints: 8 end point, 2 parallel, 1 horizontal, 1 perpendicular, 1 point on line
extrude "Extrusion20" add sketch "Sketch20" against normal up to surface (5.08 mm away)
sketch "Sketch21" plane through (101.6, 50.8, -7.0632) normal (0, 1, 0) x (1, 0, 0)
  line L0 (5.08, 0) -> (-63.5, -17.145) projected
  line L1 (0, -1.27) -> (0, 0) projected
  line L2 (5.08, 0) -> (0, -1.27)
  line L3 (0, -1.27) -> (0, 0)
  line L4 (0, -1.27) -> (0, 0)
  line L5 (0, 0) -> (5.08, 0) projected
  line L6 (5.08, 0) -> (0, 0)
  point P0 (-101.6, -7.0632)
  constraints: 8 end point, 2 collinear, 1 vertical
extrude "Extrusion21" cut sketch "Sketch21" against normal up to surface (6.35 mm away)
sketch "Sketch22" plane through (-104.775, -6.35, -50.8) normal (-1, 0, 0) x (0, 0, 1)
  line L0 (101.6, 50.8) -> (100.0125, 50.8) projected
  line L1 (0, 6.35) -> (101.6, 6.35)
  line L2 (101.6, 6.35) -> (101.6, 50.8)
  line L3 (101.6, 50.8) -> (0, 50.8)
  line L4 (0, 50.8) -> (0, 6.35)
  line L5 (0, 28.575) -> (101.6, 28.575)
  line L6 (50.8, 6.35) -> (50.8, 50.8)
  line L7 (102.87, 5.08) -> (-1.27, 5.08)
  line L8 (-1.27, 5.08) -> (-1.27, 52.07)
  line L9 (-1.27, 52.07) -> (102.87, 52.07)
  line L10 (102.87, 52.07) -> (102.87, 5.08)
  line L11 (102.87, 5.08) -> (-1.27, 52.07) construction
  line L12 (-1.27, 5.08) -> (102.87, 52.07) construction
  point P0 (50.8, 28.575)
  dimension "d127" = 104.14
  dimension "d128" = 46.99
  constraints: 24 end point, 6 midpoint, 4 parallel, 2 horizontal, 2 perpendicular
  measures "d127" distance of L8.end L9.end
  measures "d128" distance of L7.end L8.end
extrude "Extrusion22" cut sketch "Sketch22" against normal blind 194.945 contours L2 L5 L6 L3 L0 | L2 L1 L6 L5 | L6 L5 L4 L3 | L6 L1 L4 L5 | L7 L8 L9 L10
sketch "Sketch23" plane through (90.17, -6.35, -50.8) normal (-1, 0, 0) x (0, 0, 1)
  line L0 (0, -5.08) -> (0, 50.8) projected
  line L1 (0, 6.35) -> (101.4986, 6.35)
  line L2 (101.4986, 6.35) -> (101.4986, 50.8)
  line L3 (101.4986, 50.8) -> (0, 50.8)
  line L4 (0, 50.8) -> (0, 6.35)
  line L5 (102.7686, 5.08) -> (-1.27, 5.08)
  line L6 (-1.27, 5.08) -> (-1.27, 52.07)
  line L7 (-1.27, 52.07) -> (102.7686, 52.07)
  line L8 (102.7686, 52.07) -> (102.7686, 5.08)
  line L9 (-1.27, 28.575) -> (102.7686, 28.575)
  line L10 (94.0747, 52.07) -> (89.9498, 5.08)
  line L11 (89.9498, 5.08) -> (102.7686, 5.08)
  line L12 (102.7686, 52.07) -> (102.7686, 5.08)
  line L13 (102.7686, 52.07) -> (94.0747, 52.07)
  point P0 (50.8, 6.35)
  point P1 (92.0122, 28.575)
  dimension "d131" = 1.27
  constraints: 26 end point, 4 parallel, 3 perpendicular, 3 point on line, 2 collinear, 2 midpoint, 1 horizontal, 3 other
  measures "d131" distance between parallel lines of L1 L5
extrude "Extrusion23" cut sketch "Sketch23" against normal up to surface (11.43 mm away) contours L5 L6 L9 L0 | L0 L1 L10 L5 | L0 L9 L10 L1 | L10 L1 L2 L9 L8 L5 | L10 L9 L2 L1 | L10 L3 L2 L9 | L9 L2 L3 L10 L7 L8
sketch "Sketch24" plane through (-98.425, 6.35, 62.23) normal (0, 0, 1) x (1, 0, 0)
  line L0 (-6.35, 6.35) -> (-6.35, -12.7) projected
  line L1 (-6.35, 25.4) -> (21.5279, 25.4) projected
  line L2 (-6.35, 6.35) -> (0, 6.35)
  line L3 (0, 6.35) -> (0, 25.4)
  line L4 (0, 25.4) -> (-6.35, 25.4)
  line L5 (-6.35, 25.4) -> (-6.35, 6.35)
  point P0 (98.425, -6.35)
  dimension "d134" = 6.35
  constraints: 8 end point, 2 parallel, 1 horizontal, 1 perpendicular, 1 point on line
  measures "d134" distance of L4.end L3.end
extrude "Extrusion24" add sketch "Sketch24" against normal up to surface (5.08 mm away)
sketch "Sketch25" plane through (88.9, -6.35, -44.45) normal (0, 1, 0) x (1, 0, 0)
  line L0 (-32.6749, -6.35) -> (-154.6501, -6.35) projected
  line L1 (-154.6501, -6.35) -> (-193.675, -6.35)
  line L2 (-193.675, -101.6) -> (-193.675, 6.35) projected
  line L3 (-93.6625, -37.3278) -> (-32.6749, -6.35) projected
  line L4 (-32.6749, -6.35) -> (12.7, -6.35)
  line L5 (12.7, -101.6) -> (12.7, 6.35) projected
  line L6 (-193.675, 6.35) -> (12.7, 6.35) projected
  line L7 (-193.675, -6.35) -> (12.7, -6.35)
  line L8 (12.7, -6.35) -> (12.7, 6.35)
  line L9 (12.7, 6.35) -> (-193.675, 6.35)
  line L10 (-193.675, 6.35) -> (-193.675, -6.35)
  line L11 (-193.675, 0) -> (12.7, 0)
  line L12 (-6.35, -81.677) -> (-6.35, -7.223) projected
  line L13 (-6.35, -7.223) -> (-6.35, -6.35)
  line L14 (-32.6749, -6.35) -> (-6.35, -6.35)
  line L15 (-19.5125, -6.35) -> (-19.5125, 6.35)
  line L16 (-180.975, -7.223) -> (-180.975, -81.677) projected
  line L17 (-180.975, -7.223) -> (-180.975, -6.35)
  line L18 (-180.975, -6.35) -> (-154.6501, -6.35)
  line L19 (-167.8125, -6.35) -> (-167.8125, 6.35)
  circle A0 centre (-167.8125, 0) radius 2.667
  circle A1 centre (-19.5125, 0) radius 2.667
  circle A2 centre (-93.6625, -44.45) radius 2.54 projected
  circle A3 centre (-143.6687, -69.85) radius 2.54 projected
  line L20 (-93.6625, -44.45) -> (-143.6687, -69.85)
  circle A4 centre (-43.6562, -69.85) radius 2.54 projected
  line L21 (-93.6625, -44.45) -> (-43.6562, -69.85)
  circle A5 centre (-118.6656, -57.15) radius 2.667
  circle A6 centre (-68.6594, -57.15) radius 2.667
  point P0 (-88.9, -44.45)
  dimension "d137" = 5.334
  dimension "d138" = 5.334
  dimension "d139" = 5.334
  dimension "d140" = 5.334
  constraints: 30 end point, 8 midpoint, 7 point on line, 4 centre point, 4 perpendicular, 2 collinear, 2 horizontal, 2 parallel, 1 vertical
  measures "d137" diameter of A0
  measures "d138" diameter of A1
  measures "d139" diameter of A5
  measures "d140" diameter of A6
extrude "Extrusion25" cut sketch "Sketch25" against normal blind 25.4 contours A1 L11 L15 | L15 L11 A1 | A0 L11 L19 | L19 L11 A0 | L15 A1 L11 | L11 A1 L15 | L19 A0 L11 | L11 A0 L19 | A5 L20 | L20 A5 | A6 L21 | L21 A6
sketch "Sketch26" plane through (-44.45, 55.88, 12.7) normal (0, 1, 0) x (1, 0, 0)
  line L0 (-60.325, -44.45) -> (146.05, -44.45) projected
  line L1 (-44.45, -24.765) -> (-57.0686, -44.45) projected
  line L2 (-60.325, -44.45) -> (-44.45, -24.765)
  line L3 (-60.325, -49.53) -> (-36.4641, -49.53) projected
  line L4 (-44.45, -24.765) -> (-60.325, -49.53)
  line L5 (-60.325, -49.53) -> (-60.325, -44.45)
  point P0 (44.45, 12.7)
  constraints: 6 end point, 1 point on line, 1 vertical
extrude "Extrusion26" add sketch "Sketch26" against normal up to surface (5.08 mm away)
sketch "Sketch27" plane through (87.6387, 50.8, 57.15) normal (0, 1, 0) x (1, 0, 0)
  line L0 (0, 0) -> (1.3708, 0) projected
  line L1 (0, 0) -> (1.3708, 0)
  line L2 (1.3723, -0.7429) -> (-49.5387, 26.8205) projected
  line L3 (1.3708, 0) -> (1.3723, -0.7429)
  line L4 (1.3723, -0.7429) -> (0, 0)
  point P0 (-87.6387, 57.15)
  constraints: 6 end point, 1 collinear, 1 horizontal
extrude "Extrusion27" add sketch "Sketch27" along normal up to surface (5.08 mm away)
sketch "Sketch28" plane through (106.68, 29.3688, -0.7937) normal (1, 0, 0) x (0, 0, -1)
  line L0 (6.2694, 15.0813) -> (6.2694, 26.5113) projected
  line L1 (6.2694, 15.0813) -> (-63.0237, 15.0813)
  line L2 (-63.0237, -40.7988) -> (-63.0237, 26.5113) projected
  line L3 (5.738, 21.4312) -> (-38.2588, 21.4312) projected
  line L4 (-0.7937, 21.4312) -> (-0.7937, 15.0813)
  line L5 (-39.8044, 21.4312) -> (-39.8044, 26.5113) projected
  line L6 (-39.8044, 21.4312) -> (-39.8044, 15.0813)
  line L7 (-39.8044, 21.4312) -> (-0.7937, 21.4312)
  line L8 (-4.6458, 26.5113) -> (-11.8827, 26.5113) projected
  point P0 (-0.7937, -29.3688)
  point P1 (-38.2588, 21.4312)
  constraints: 8 end point, 4 point on line, 2 perpendicular, 1 horizontal, 1 parallel
extrude "Extrusion28" cut sketch "Sketch28" against normal blind 5.08
body "Solid1"
